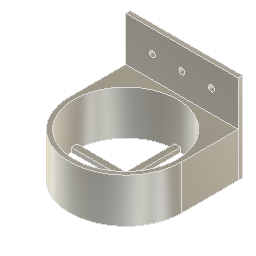
Держатль под балоны (Autodesk Fusion 360 design; units mm, degrees)
Autodesk Fusion 360 part; units mm, degrees
sketch "Sketch1" plane through (0, 0, 0) normal (0, 0, 1) x (1, 0, 0)
  circle A0 centre (0, 0) radius 35
  circle A1 centre (0, 0) radius 38
  line L0 (-38, 0) -> (-38, 38)
  line L1 (-38, 38) -> (0, 38)
  line L2 (0, 1.75) -> (0, 22.5)
  line L3 (38, 38) -> (0, 38)
  line L4 (38, 0) -> (38, 38)
  line L5 (2.0599, 34.9393) -> (2.0599, 2)
  line L6 (2.0599, -2) -> (2.0599, -34.9393)
  line L7 (-34.9428, 2) -> (-1.9401, 2)
  line L8 (2.0599, 2) -> (34.9428, 2)
  line L9 (-1.9401, 34.9462) -> (-1.9401, 2)
  line L10 (-1.9401, -2) -> (-1.9401, -34.9462)
  line L11 (-34.9428, -2) -> (-1.9401, -2)
  line L12 (2.0599, -2) -> (34.9428, -2)
  dimension "d1" = 70
  dimension "d2" = 3
  dimension "d27" = 38
  dimension "d28" = 38
  constraint coincident A0.centre A1.centre
  constraint coincident A1 L0.start
  constraint vertical L0
  constraint perpendicular L0 L1
  constraint symmetric L0.start L2 L4.start
  constraint symmetric L0.end L2 L3.start
  constraint coincident A1 L1.end
  constraint coincident A0 L5.start
  constraint coincident A0 L9.start
  constraint coincident A0 L10.end
  constraint coincident A0 L6.end
  constraint coincident A0 L11.start
  constraint coincident A0 L7.start
  constraint coincident A0 L12.end
  constraint coincident A0 L8.end
  constraint coincident L5.end L7
  constraint coincident L6.start L11
  constraint collinear L5 L6
  constraint collinear L7 L8
  constraint collinear L9 L10
  constraint collinear L11 L12
  measures "d1" diameter of A0
  measures "d27" distance of A0.centre L0
  measures "d28" distance of A0.centre L1
extrude "Extrude1" add sketch "Sketch1" along normal blind 3 contours A0 L5 L6 L7 L8 L9 L10 L11 L12 | A1 | A1 L3 L4 | A1 L0 L1
sketch "Sketch3" plane through (0, 38, 0) normal (0, 1, 0) x (-1, 0, 0)
  line L0 (-38, 0) -> (38, 0)
  line L1 (38, 0) -> (38, 3)
  line L2 (38, 3) -> (-38, 3)
  line L3 (-38, 0) -> (38, 0)
  line L4 (38, 0) -> (38, 60)
  line L5 (38, 60) -> (0, 60)
  circle A0 centre (-20, 45) radius 2
  circle A1 centre (0, 45) radius 2
  circle A2 centre (20, 45) radius 2
  line L6 (-38, 60) -> (0, 60)
  line L7 (-38, 0) -> (-38, 60)
  line L8 (-38, 0) -> (38, 0)
  line L9 (-38, 3) -> (-38, 0)
  dimension "d9" = 60
  dimension "d10" = 38
  dimension "d11" = 4
  constraint horizontal L3
  constraint vertical L4
  constraint horizontal L5
  constraint coincident L0.start L3.start
  constraint coincident L0.end L1.start
  measures "d9" distance of L0.end L4.end
  measures "d10" distance of L4.end L5.end
  measures "d11" diameter of A2
extrude "Extrude4" add sketch "Sketch3" along normal blind 3
extrude "Extrude5" add sketch "Sketch1" along normal blind 30
